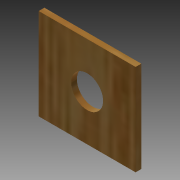
# Autodesk Inventor part: segment0b
Saved by Autodesk Inventor 2013 (Build 170138000, 138)
## iProperties
Created: 2014-10-12
Part Number: segment0b
Material: Plywood, Finish
Document SubType Name: Modeling
Designer: Masta
Density: 1 g/cm^3
Author: Masta
Autodesk Inventor part; units mm, degrees
ref_plane "YZ Plane" through (0, 0, 0) normal (1, 0, 0) x (0, 1, 0)
ref_plane "XZ Plane" through (0, 0, 0) normal (0, 1, 0) x (-1, 0, 0)
ref_plane "XY Plane" through (0, 0, 0) normal (0, 0, 1) x (1, 0, 0)
sketch "Sketch1" plane through (0, 0, 0) normal (0, 1, 0) x (-1, 0, 0)
  line L0 (-42.5, -40) -> (42.5, -40)
  line L1 (42.5, -40) -> (42.5, 40)
  line L2 (42.5, 40) -> (-42.5, 40)
  line L3 (-42.5, 40) -> (-42.5, -40)
  line L4 (-42.5, -40) -> (42.5, 40) construction
  line L5 (42.5, -40) -> (-42.5, 40) construction
  circle A0 centre (0, 0) radius 14
  dimension "d0" = 85
  dimension "d1" = 80
  dimension "d4" = 28
  constraints: 12 end point, 2 midpoint, 2 parallel, 1 centre point, 1 coincident, 1 horizontal, 1 perpendicular
  measures "d0" distance of L2.end L1.end
  measures "d1" distance of L1.end L0.end
  measures "d4" diameter of A0
extrude "Extrusion1" add sketch "Sketch1" along normal blind 5
body "Solid1"
